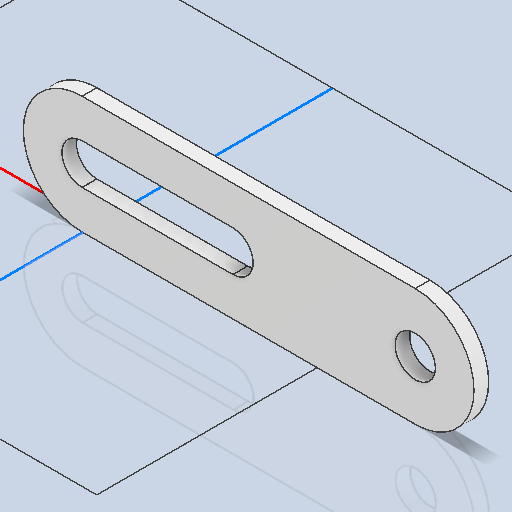
# Autodesk Inventor part: Hardstop Gusset
Saved by Autodesk Inventor 2026 (Build 300175000, 175)
## iProperties
Created: 2025-04-12
Part Number: Hardstop Gusset
Material: Acetal Resin, White
Document SubType Name: Modeling
Designer: avere
Density: 1.425 g/cm^3
Appearance: Smooth - White
Author: avere
Autodesk Inventor part; units mm, degrees
ref_plane "YZ Plane" through (0, 0, 0) normal (1, 0, 0) x (0, 1, 0)
ref_plane "XZ Plane" through (0, 0, 0) normal (0, 1, 0) x (-1, 0, 0)
ref_plane "XY Plane" through (0, 0, 0) normal (0, 0, 1) x (1, 0, 0)
sketch "main" plane through (0, 0, 0) normal (0, 0, 1) x (1, 0, 0)
  circle A0 centre (20.1021, 1.4076) radius 2.1844
  arc A1 (-15.8903, 3.592) -> (-15.8903, -0.7768) centre (-15.8903, 1.4076) ccw
  arc A2 (20.1021, -4.9424) -> (20.1021, 7.7576) centre (20.1021, 1.4076) ccw
  arc A3 (-15.8903, 7.7576) -> (-15.8903, -4.9424) centre (-15.8903, 1.4076) ccw
  line L0 (-15.8903, 7.7576) -> (20.1021, 7.7576)
  line L1 (20.1021, -4.9424) -> (-15.8903, -4.9424)
  arc A4 (0.4077, -0.7768) -> (0.4077, 3.592) centre (0.4077, 1.4076) ccw
  line L2 (-15.8903, 3.592) -> (0.4077, 3.592)
  line L3 (0.4077, -0.7768) -> (-15.8903, -0.7768)
  point P0 (-1.0706, 1.6197)
  dimension "d0" = 12.7
  dimension "d1" = 12.7
  dimension "d3" = 35.9924
  dimension "d4" = 4.3688
  dimension "d5" = 4.3688
  measures "d0" diameter of A2
  measures "d1" diameter of A3
  measures "d3" distance of A0.centre A1.centre
  measures "d4" diameter of A4
  measures "d5" diameter of A1
sketch "Sketch1" plane through (0, 0, 0) normal (0, 0, 1) x (1, 0, 0)
  circle A0 centre (35.9924, 0) radius 2.1844
  arc A1 (0, 2.1844) -> (0, -2.1844) centre (0, 0) ccw
  arc A2 (35.9924, -6.35) -> (35.9924, 6.35) centre (35.9924, 0) ccw
  arc A3 (0, 6.35) -> (0, -6.35) centre (0, 0) ccw
  line L0 (0, 6.35) -> (35.9924, 6.35)
  line L1 (35.9924, -6.35) -> (0, -6.35)
  arc A4 (16.298, -2.1844) -> (16.298, 2.1844) centre (16.298, 0) ccw
  line L2 (0, 2.1844) -> (16.298, 2.1844)
  line L3 (16.298, -2.1844) -> (0, -2.1844)
  constraints: 1 other
extrude "Extrusion1" add sketch "Sketch1" along normal blind 1.5875
body "Solid1"
